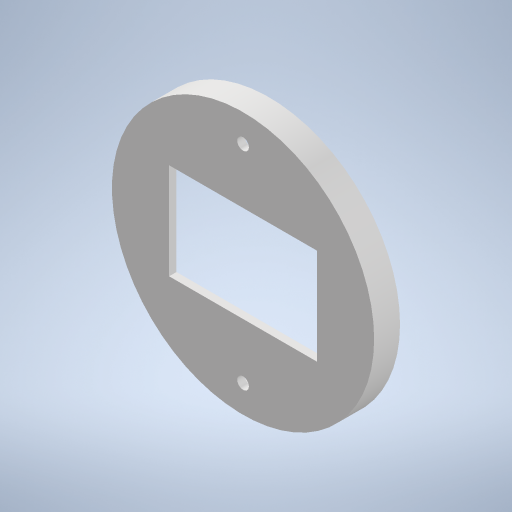
# Autodesk Inventor part: LensMount_frame
Saved by Autodesk Inventor 2023 (Build 270158000, 158)
## iProperties
Created: 2022-10-31
Part Number: LensMount_frame
Material: Generic
Document SubType Name: Modeling
Designer: Piotr
Density: 1 g/cm^3
Appearance: Default
Author: Piotr
Autodesk Inventor part; units mm, degrees
ref_plane "YZ Plane" through (0, 0, 0) normal (1, 0, 0) x (0, 1, 0)
ref_plane "XZ Plane" through (0, 0, 0) normal (0, 1, 0) x (-1, 0, 0)
ref_plane "XY Plane" through (0, 0, 0) normal (0, 0, 1) x (1, 0, 0)
sketch "Sketch1" plane through (0, 0, 0) normal (0, 0, 1) x (1, 0, 0)
  circle A0 centre (0, 0) radius 34 construction
  circle A1 centre (0, 28) radius 1.6 projected
  circle A2 centre (0, -28) radius 1.6 projected
  circle A3 centre (0, 0) radius 34.25
  circle A4 centre (0, 0) radius 35.45
  dimension "d0" = 0.25
  dimension "d1" = 1.2
  constraints: 2 centre point
  measures "d0" radial gap between concentric circles of A0 A3
  measures "d1" radial gap between concentric circles of A3 A4
extrude "Extrusion1" add sketch "Sketch1" against normal blind 5 contours A4
sketch "Sketch4" plane through (0, 0, 0) normal (0, 0, 1) x (1, 0, 0)
  circle A0 centre (0, 0) radius 35.45 projected
  circle A1 centre (0, 28) radius 1.6 projected
  circle A2 centre (0, -28) radius 1.6 projected
extrude "Extrusion2" add sketch "Sketch4" along normal blind 2
sketch "Sketch5" plane through (0, 0, 2) normal (0, 0, 1) x (1, 0, 0)
  circle A0 centre (0, 0) radius 35.45 projected
  line L0 (-20, 13) -> (20, 13)
  line L1 (20, 13) -> (20, -13)
  line L2 (20, -13) -> (-20, -13)
  line L3 (-20, -13) -> (-20, 13)
  line L4 (-20, 13) -> (20, -13) construction
  line L5 (20, 13) -> (-20, -13) construction
  dimension "d6" = 40
  dimension "d7" = 26
  constraints: 12 end point, 2 midpoint, 2 parallel, 1 horizontal, 1 perpendicular
  measures "d6" distance of L1.end L2.end
  measures "d7" distance of L0.end L1.end
extrude "Extrusion3" cut sketch "Sketch5" against normal through all contours L0 L1 L2 L3
body "Solid1"
